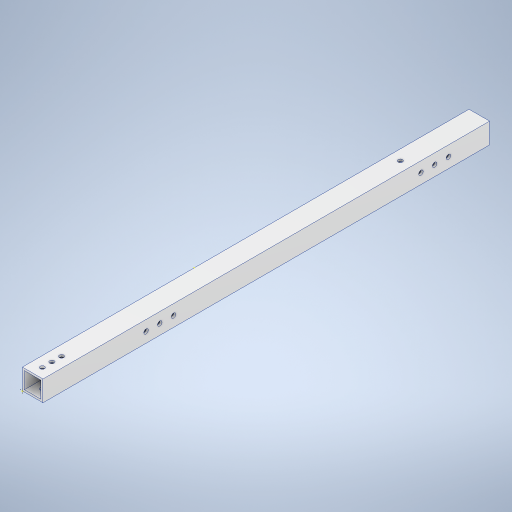
# Autodesk Inventor part: 射出_角柱5
Saved by Autodesk Inventor 2023 (Build 270158000, 158)
## iProperties
Created: 2022-04-20
Part Number: 射出_角柱5
Material: アルミニウム 6061
Document SubType Name: Modeling
Designer: yuta
Density: 2.7 g/cm^3
Appearance: アルミニウム - フラット
Mass: 70.4912 g
Surface Area: 352.439 cm^2
Volume: 26.1079 cm^3
Author: yuta
Autodesk Inventor part; units mm, degrees
ref_plane "YZ Plane" through (0, 0, 0) normal (1, 0, 0) x (0, 1, 0)
ref_plane "XZ Plane" through (0, 0, 0) normal (0, 1, 0) x (-1, 0, 0)
ref_plane "XY Plane" through (0, 0, 0) normal (0, 0, 1) x (1, 0, 0)
sketch "スケッチ1" plane through (0, 0, 0) normal (0, 0, 1) x (1, 0, 0)
  line L0 (0, 0) -> (15, 0)
  line L1 (15, 0) -> (15, 15)
  line L2 (15, 15) -> (0, 15)
  line L3 (0, 15) -> (0, 0)
  dimension "d0" = 15
  dimension "d1" = 15
  constraints: 8 end point, 2 parallel, 1 horizontal, 1 perpendicular
  measures "d0" distance of L2.end L1.end
  measures "d1" distance of L1.end L0.end
extrude "押し出し1" add sketch "スケッチ1" along normal blind 140
sketch "スケッチ3" plane through (0, 0, 0) normal (0, 0, -1) x (-1, 0, 0)
  line L0 (0, 0) -> (-15, 0)
  line L1 (-15, 0) -> (-15, 15)
  line L2 (-15, 15) -> (0, 15)
  line L3 (0, 15) -> (0, 0)
  dimension "d18" = 15
  dimension "d19" = 15
  constraints: 8 end point, 2 parallel, 1 horizontal, 1 perpendicular
  measures "d18" distance of L1.end L2.end
  measures "d19" distance of L0.end L1.end
extrude "押し出し2" add sketch "スケッチ3" along normal blind 200
sketch "スケッチ4" plane through (0, 0, -200) normal (0, 0, -1) x (-1, 0, 0)
  point P0 (0, 0)
sketch "スケッチ6" plane through (0, 0, 140) normal (0, 0, 1) x (1, 0, 0)
  line L0 (0, 0) -> (0, 15) projected
  line L1 (15, 15) -> (15, 0) projected
  line L2 (0, 0) -> (15, 0)
  line L3 (15, 0) -> (15, 15)
  line L4 (15, 15) -> (0, 15)
  line L5 (0, 15) -> (0, 0)
  constraints: 8 end point, 2 parallel, 1 horizontal, 1 perpendicular
extrude "押し出し3" cut sketch "スケッチ6" against normal blind 15
sketch "スケッチ7" plane through (0, 0, 125) normal (0, 0, 1) x (1, 0, 0)
  point P0 (0, 0)
  point P1 (0, 0)
  constraints: 1 coincident
sketch "スケッチ8" plane through (0, 0, -200) normal (-1, 0, 0) x (0, 0, 1)
  circle A0 centre (240, 7.5) radius 1.6
  line L0 (0, 15) -> (325, 15) projected
  line L1 (325, 0) -> (325, 15) projected
  point P0 (200, 0)
  dimension "d34" = 3.2
  dimension "d35" = 7.5
  dimension "d36" = 85
  constraints: 1 centre point
  measures "d34" diameter of A0
  measures "d35" distance from line of L0 A0.centre
  measures "d36" distance from line of L1 A0.centre
hole "穴3" at (0, 7.5, 40) direction (1, 0, 0) diameter 3.2 end through all
sketch "スケッチ9" plane through (0, 0, -200) normal (-1, 0, 0) x (0, 0, 1)
  circle A0 centre (250, 7.5) radius 1.6
  line L0 (0, 0) -> (325, 0) projected
  line L1 (325, 0) -> (325, 15) projected
  circle A1 centre (230, 7.5) radius 1.6
  point P0 (200, 0)
  dimension "d44" = 3.2
  dimension "d45" = 7.5
  dimension "d46" = 75
  dimension "d47" = 3.2
  dimension "d48" = 7.5
  dimension "d49" = 20
  constraints: 2 centre point
  measures "d44" diameter of A0
  measures "d45" distance from line of L0 A0.centre
  measures "d46" distance from line of L1 A0.centre
  measures "d47" diameter of A1
  measures "d48" distance from line of L0 A1.centre
  measures "d49" distance of A0.centre A1.centre
hole "穴4" at (0, 7.5, 30) at (0, 7.5, 50) direction (1, 0, 0) diameter 3.2 end through all
sketch "スケッチ10" plane through (0, 15, -200) normal (0, 1, 0) x (1, 0, 0)
  circle A0 centre (7.5, -318) radius 1.6
  line L0 (0, 0) -> (0, -325) projected
  line L1 (0, -325) -> (15, -325) projected
  circle A1 centre (7.5, -311) radius 1.6
  circle A2 centre (7.5, -304) radius 1.6
  point P0 (0, -200)
  dimension "d57" = 3.2
  dimension "d58" = 7.5
  dimension "d59" = 7
  dimension "d60" = 3.2
  dimension "d61" = 3.2
  dimension "d62" = 7
  dimension "d63" = 7
  constraints: 3 centre point
  measures "d57" diameter of A0
  measures "d58" distance from line of L0 A0.centre
  measures "d59" distance from line of L1 A0.centre
  measures "d60" diameter of A1
  measures "d61" diameter of A2
  measures "d62" distance of A1.centre A0.centre
  measures "d63" distance of A2.centre A1.centre
hole "穴5" at (7.5, 15, 104) at (7.5, 15, 111) at (7.5, 15, 118) direction (0, -1, 0) diameter 3.2 end through all
sketch "スケッチ11" plane through (15, 0, -200) normal (1, 0, 0) x (0, 0, -1)
  line L0 (0, 15) -> (0, 0) projected
  line L1 (-325, 0) -> (0, 0) projected
  point P0 (-200, 0)
  point P1 (-30, 7.5)
  point P2 (-40, 7.5)
  point P3 (-50, 7.5)
  dimension "d71" = 30
  dimension "d72" = 7.5
  dimension "d73" = 10
  dimension "d74" = 10
  measures "d71" distance from line of L0 point (-30, 7.5)
  measures "d72" distance from line of L1 point (-30, 7.5)
  measures "d73" distance of point (-40, 7.5) point (-30, 7.5)
  measures "d74" distance of point (-50, 7.5) point (-40, 7.5)
hole "穴6" at (15, 7.5, -150) at (15, 7.5, -160) at (15, 7.5, -170) direction (-1, 0, 0) diameter 3.2 end through all
sketch "スケッチ12" plane through (0, 0, 125) normal (0, 0, 1) x (1, 0, 0)
  line L0 (1.5, 13.5) -> (13.5, 13.5)
  line L1 (13.5, 13.5) -> (13.5, 1.5)
  line L2 (13.5, 1.5) -> (1.5, 1.5)
  line L3 (1.5, 1.5) -> (1.5, 13.5)
  line L4 (0, 15) -> (15, 15) projected
  line L5 (0, 0) -> (0, 15) projected
  dimension "d82" = 12
  dimension "d83" = 12
  dimension "d84" = 1.5
  dimension "d85" = 1.5
  constraints: 8 end point, 2 parallel, 1 horizontal, 1 perpendicular
  measures "d82" distance of L1.end L2.end
  measures "d83" distance of L0.end L1.end
  measures "d84" distance between parallel lines of L4 L0
  measures "d85" distance between parallel lines of L5 L3
extrude "押し出し4" cut sketch "スケッチ12" against normal blind 450
sketch "スケッチ13" plane through (0, 15, -200) normal (0, 1, 0) x (1, 0, 0)
  point P0 (0, -200)
sketch "スケッチ14" plane through (0, 15, -200) normal (0, 1, 0) x (1, 0, 0)
  line L0 (15, 0) -> (15, -325) projected
  line L1 (0, 0) -> (15, 0) projected
  point P0 (0, -200)
  point P1 (7.5, -57.5)
  dimension "d88" = 7.5
  dimension "d89" = 57.5
  measures "d88" distance from line of L0 point (7.5, -57.5)
  measures "d89" distance from line of L1 point (7.5, -57.5)
hole "穴7" at (7.5, 15, -142.5) direction (0, -1, 0) diameter 3.2 end through all
